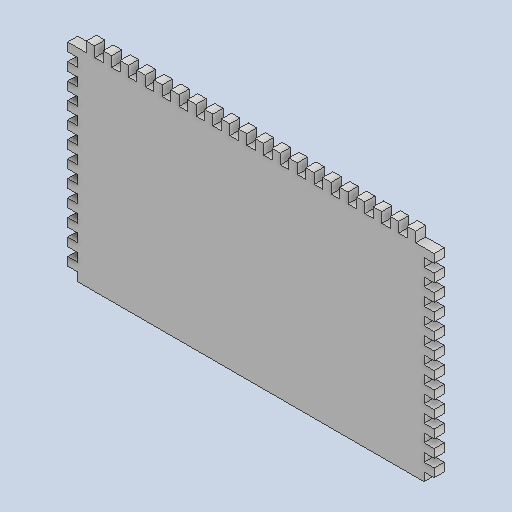
# Autodesk Inventor part: longsten
Saved by Autodesk Inventor 2022 (Build 260153000, 153)
## iProperties
Created: 2023-05-26
Part Number: longsten
Material: Типовые
Document SubType Name: Modeling
Designer: korsh624
Density: 1 g/cm^3
Appearance: По умолчанию
Author: korsh624
Autodesk Inventor part; units mm, degrees
ref_plane "YZ Plane" through (0, 0, 0) normal (1, 0, 0) x (0, 1, 0)
ref_plane "XZ Plane" through (0, 0, 0) normal (0, 1, 0) x (-1, 0, 0)
ref_plane "XY Plane" through (0, 0, 0) normal (0, 0, 1) x (1, 0, 0)
sketch "Эскиз1" plane through (0, 0, 0) normal (0, 0, 1) x (1, 0, 0)
  line L0 (-190, 0) -> (-185, 0) projected
  line L1 (-185, 0) -> (-185, 6) projected
  line L2 (-190, 6) -> (-185, 6) projected
  line L3 (-190, 0) -> (-190, 6) projected
  line L4 (-180, 0) -> (-175, 0) projected
  line L5 (-175, 0) -> (-175, 6) projected
  line L6 (-180, 6) -> (-175, 6) projected
  line L7 (-180, 0) -> (-180, 6) projected
  line L8 (-170, 0) -> (-165, 0) projected
  line L9 (-165, 0) -> (-165, 6) projected
  line L10 (-170, 6) -> (-165, 6) projected
  line L11 (-170, 0) -> (-170, 6) projected
  line L12 (-160, 0) -> (-155, 0) projected
  line L13 (-155, 0) -> (-155, 6) projected
  line L14 (-160, 6) -> (-155, 6) projected
  line L15 (-160, 0) -> (-160, 6) projected
  line L16 (-150, 0) -> (-145, 0) projected
  line L17 (-145, 0) -> (-145, 6) projected
  line L18 (-150, 6) -> (-145, 6) projected
  line L19 (-150, 0) -> (-150, 6) projected
  line L20 (-140, 0) -> (-135, 0) projected
  line L21 (-135, 0) -> (-135, 6) projected
  line L22 (-140, 6) -> (-135, 6) projected
  line L23 (-140, 0) -> (-140, 6) projected
  line L24 (-130, 0) -> (-125, 0) projected
  line L25 (-125, 0) -> (-125, 6) projected
  line L26 (-130, 6) -> (-125, 6) projected
  line L27 (-130, 0) -> (-130, 6) projected
  line L28 (-120, 0) -> (-115, 0) projected
  line L29 (-115, 0) -> (-115, 6) projected
  line L30 (-120, 6) -> (-115, 6) projected
  line L31 (-120, 0) -> (-120, 6) projected
  line L32 (-110, 0) -> (-105, 0) projected
  line L33 (-105, 0) -> (-105, 6) projected
  line L34 (-110, 6) -> (-105, 6) projected
  line L35 (-110, 0) -> (-110, 6) projected
  line L36 (-100, 0) -> (-95, 0) projected
  line L37 (-95, 0) -> (-95, 6) projected
  line L38 (-100, 6) -> (-95, 6) projected
  line L39 (-100, 0) -> (-100, 6) projected
  line L40 (-90, 0) -> (-85, 0) projected
  line L41 (-85, 0) -> (-85, 6) projected
  line L42 (-90, 6) -> (-85, 6) projected
  line L43 (-90, 0) -> (-90, 6) projected
  line L44 (-80, 0) -> (-75, 0) projected
  line L45 (-75, 0) -> (-75, 6) projected
  line L46 (-80, 6) -> (-75, 6) projected
  line L47 (-80, 0) -> (-80, 6) projected
  line L48 (-65, 0) -> (-65, 6) projected
  line L49 (-70, 0) -> (-65, 0) projected
  line L50 (-65, 0) -> (-65, 6) projected
  line L51 (-70, 6) -> (-65, 6) projected
  line L52 (-70, 0) -> (-70, 6) projected
  line L53 (-60, 0) -> (-55, 0) projected
  line L54 (-55, 0) -> (-55, 6) projected
  line L55 (-60, 6) -> (-55, 6) projected
  line L56 (-60, 0) -> (-60, 6) projected
  line L57 (-50, 0) -> (-45, 0) projected
  line L58 (-45, 0) -> (-45, 6) projected
  line L59 (-50, 6) -> (-45, 6) projected
  line L60 (-50, 0) -> (-50, 6) projected
  line L61 (-40, 0) -> (-35, 0) projected
  line L62 (-35, 0) -> (-35, 6) projected
  line L63 (-40, 6) -> (-35, 6) projected
  line L64 (-40, 0) -> (-40, 6) projected
  line L65 (-30, 0) -> (-25, 0) projected
  line L66 (-25, 0) -> (-25, 6) projected
  line L67 (-30, 6) -> (-25, 6) projected
  line L68 (-30, 0) -> (-30, 6) projected
  line L69 (-20, 0) -> (-15, 0) projected
  line L70 (-15, 0) -> (-15, 6) projected
  line L71 (-20, 6) -> (-15, 6) projected
  line L72 (-20, 0) -> (-20, 6) projected
  line L73 (-10, 0) -> (-5, 0) projected
  line L74 (-5, 0) -> (-5, 6) projected
  line L75 (-10, 6) -> (-5, 6) projected
  line L76 (-10, 0) -> (-10, 6) projected
  line L77 (0, 0) -> (5, 0) projected
  line L78 (5, 0) -> (5, 6) projected
  line L79 (0, 6) -> (5, 6) projected
  line L80 (0, 0) -> (0, 6) projected
  line L81 (5, 0) -> (10, 0) projected
  line L82 (-195, 0) -> (-190, 0) projected
  line L83 (-195, 0) -> (10, 0)
  line L84 (10, 0) -> (10, -120)
  line L85 (10, -120) -> (-195, -120)
  line L86 (-195, -120) -> (-195, 0)
  line L87 (5, 0) -> (10, 0) projected
  line L88 (-195, 0) -> (-201, 0)
  line L89 (-201, 0) -> (-201, -5)
  line L90 (-201, -5) -> (-195, -5)
  line L91 (-195, -5) -> (-195, 0)
  line L92 (-195, -15) -> (-195, -10)
  line L93 (-195, -10) -> (-201, -10)
  line L94 (-201, -10) -> (-201, -15)
  line L95 (-201, -15) -> (-195, -15)
  line L96 (-195, -25) -> (-195, -20)
  line L97 (-195, -20) -> (-201, -20)
  line L98 (-201, -20) -> (-201, -25)
  line L99 (-201, -25) -> (-195, -25)
  line L100 (-195, -35) -> (-195, -30)
  line L101 (-195, -30) -> (-201, -30)
  line L102 (-201, -30) -> (-201, -35)
  line L103 (-201, -35) -> (-195, -35)
  line L104 (-195, -45) -> (-195, -40)
  line L105 (-195, -40) -> (-201, -40)
  line L106 (-201, -40) -> (-201, -45)
  line L107 (-201, -45) -> (-195, -45)
  line L108 (-195, -55) -> (-195, -50)
  line L109 (-195, -50) -> (-201, -50)
  line L110 (-201, -50) -> (-201, -55)
  line L111 (-201, -55) -> (-195, -55)
  line L112 (-195, -65) -> (-195, -60)
  line L113 (-195, -60) -> (-201, -60)
  line L114 (-201, -60) -> (-201, -65)
  line L115 (-201, -65) -> (-195, -65)
  line L116 (-195, -75) -> (-195, -70)
  line L117 (-195, -70) -> (-201, -70)
  line L118 (-201, -70) -> (-201, -75)
  line L119 (-201, -75) -> (-195, -75)
  line L120 (-195, -85) -> (-195, -80)
  line L121 (-195, -80) -> (-201, -80)
  line L122 (-201, -80) -> (-201, -85)
  line L123 (-201, -85) -> (-195, -85)
  line L124 (-195, -95) -> (-195, -90)
  line L125 (-195, -90) -> (-201, -90)
  line L126 (-201, -90) -> (-201, -95)
  line L127 (-201, -95) -> (-195, -95)
  line L128 (-195, -105) -> (-195, -100)
  line L129 (-195, -100) -> (-201, -100)
  line L130 (-201, -100) -> (-201, -105)
  line L131 (-201, -105) -> (-195, -105)
  line L132 (-195, -115) -> (-195, -110)
  line L133 (-195, -110) -> (-201, -110)
  line L134 (-201, -110) -> (-201, -115)
  line L135 (-201, -115) -> (-195, -115)
  line L136 (10, 0) -> (16, 0)
  line L137 (16, 0) -> (16, -5)
  line L138 (16, -5) -> (10, -5)
  line L139 (10, -5) -> (10, 0)
  line L140 (10, -15) -> (10, -10)
  line L141 (10, -10) -> (16, -10)
  line L142 (16, -15) -> (10, -15)
  line L143 (16, -10) -> (16, -15)
  line L144 (10, -25) -> (10, -20)
  line L145 (10, -20) -> (16, -20)
  line L146 (16, -25) -> (10, -25)
  line L147 (16, -20) -> (16, -25)
  line L148 (10, -35) -> (10, -30)
  line L149 (10, -30) -> (16, -30)
  line L150 (16, -35) -> (10, -35)
  line L151 (16, -30) -> (16, -35)
  line L152 (10, -45) -> (10, -40)
  line L153 (10, -40) -> (16, -40)
  line L154 (16, -45) -> (10, -45)
  line L155 (16, -40) -> (16, -45)
  line L156 (10, -55) -> (10, -50)
  line L157 (10, -50) -> (16, -50)
  line L158 (16, -55) -> (10, -55)
  line L159 (16, -50) -> (16, -55)
  line L160 (10, -65) -> (10, -60)
  line L161 (10, -60) -> (16, -60)
  line L162 (16, -65) -> (10, -65)
  line L163 (16, -60) -> (16, -65)
  line L164 (10, -75) -> (10, -70)
  line L165 (10, -70) -> (16, -70)
  line L166 (16, -75) -> (10, -75)
  line L167 (16, -70) -> (16, -75)
  line L168 (10, -85) -> (10, -80)
  line L169 (10, -80) -> (16, -80)
  line L170 (16, -85) -> (10, -85)
  line L171 (16, -80) -> (16, -85)
  line L172 (10, -95) -> (10, -90)
  line L173 (10, -90) -> (16, -90)
  line L174 (16, -95) -> (10, -95)
  line L175 (16, -90) -> (16, -95)
  line L176 (10, -105) -> (10, -100)
  line L177 (10, -100) -> (16, -100)
  line L178 (16, -105) -> (10, -105)
  line L179 (16, -100) -> (16, -105)
  line L180 (10, -115) -> (10, -110)
  line L181 (10, -110) -> (16, -110)
  line L182 (16, -115) -> (10, -115)
  line L183 (16, -110) -> (16, -115)
  dimension "d2" = 120
  dimension "d3" = 6
  dimension "d4" = 5
  dimension "d7" = 10
  dimension "d12" = 6
  dimension "d13" = 5
  dimension "d16" = 10
  constraints: 194 end point, 88 vertical alignment, 48 parallel, 44 collinear, 3 horizontal, 2 perpendicular, 9 other
  measures "d2" distance of L85.end L82.start
  measures "d3" distance of L90.end L89.end
  measures "d4" distance of L89.end L88.end
  measures "d7" distance of L90.end L92.start
  measures "d12" distance of L137.end L138.end
  measures "d13" distance of L136.end L137.end
  measures "d16" distance of L136.start L140.end
extrude "Выдавливание1" add sketch "Эскиз1" along normal blind 6
